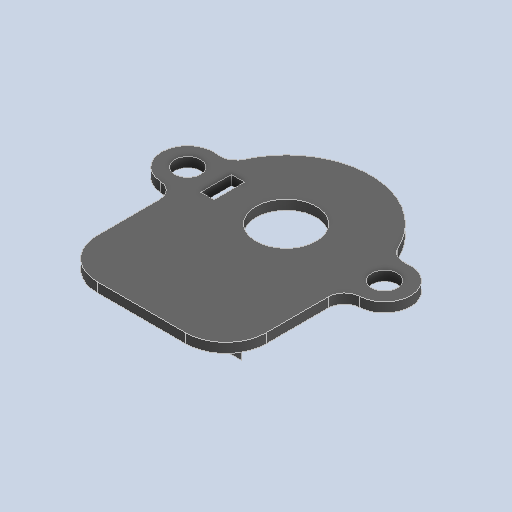
# Autodesk Inventor part: volume_case_upper
Saved by Autodesk Inventor 2026.1 (Build 301233020, 233B)
## iProperties
Created: 2026-02-01
Part Number: volume_case_upper
Material: 一般
Document SubType Name: Modeling
Designer: hibik
Density: 1 g/cm^3
Appearance: 既定
Author: hibik
Autodesk Inventor part; units mm, degrees
ref_plane "YZ Plane" through (0, 0, 0) normal (1, 0, 0) x (0, 1, 0)
ref_plane "XZ Plane" through (0, 0, 0) normal (0, 1, 0) x (-1, 0, 0)
ref_plane "XY Plane" through (0, 0, 0) normal (0, 0, 1) x (1, 0, 0)
sketch "スケッチ1" plane through (0, 0, 0) normal (0, 1, 0) x (-1, 0, 0)
  circle A0 centre (0, 0) radius 10.5
  dimension "d0" = 21
  constraints: 1 centre point, 1 coincident
  measures "d0" diameter of A0
extrude "押し出し1" add sketch "スケッチ1" along normal blind 1.2
sketch "スケッチ2" plane through (0, 1.2, 0) normal (0, 1, 0) x (1, 0, 0)
  circle A0 centre (-12.25, 0) radius 1.3 construction
  circle A1 centre (12.25, 0) radius 1.3 construction
  line L0 (15.3423, -1) -> (20.8147, -1) projected
  arc A2 (12.1791, -16.9092) -> (20.8147, -1) centre (0, 0) ccw projected
  line L1 (12.1791, -16.9092) -> (10.5, -14.0307) projected
  line L2 (10.5, -14.0307) -> (10.5, -5.244) projected
  arc A3 (12.4048, -3.2463) -> (10.5, -5.244) centre (12.5, -5.244) ccw projected
  arc A4 (12.4048, -3.2463) -> (15.3423, -1) centre (12.25, 0) ccw projected
  line L3 (9, 0) -> (9, -16.5) projected
  line L4 (-2.5, -16.5) -> (-9, -16.5) projected
  line L5 (-9, -16.5) -> (-9, 0) projected
  arc A5 (9, 0) -> (-9, 0) centre (0, 0) ccw projected
  arc A6 (15.3423, 1) -> (11.7099, 3.2048) centre (12.25, 0) ccw projected
  arc A7 (9.5571, 4.3487) -> (11.7099, 3.2048) centre (11.3776, 5.177) ccw projected
  arc A8 (9.5571, 4.3487) -> (9.333, 4.811) centre (0, 0) ccw projected
  line L6 (9.333, 4.811) -> (18.2916, 9.9833) projected
  arc A9 (20.8147, 1) -> (18.2916, 9.9833) centre (0, 0) ccw projected
  line L7 (20.8147, 1) -> (15.3423, 1) projected
  line L8 (-10.5, -5.244) -> (-10.5, -14.0307) projected
  line L9 (-12.1791, -16.9092) -> (-10.5, -14.0307) projected
  arc A10 (-20.8147, -1) -> (-12.1791, -16.9092) centre (0, 0) ccw projected
  line L10 (-15.3423, -1) -> (-20.8147, -1) projected
  arc A11 (-15.3423, -1) -> (-12.4048, -3.2463) centre (-12.25, 0) ccw projected
  arc A12 (-10.5, -5.244) -> (-12.4048, -3.2463) centre (-12.5, -5.244) ccw projected
  arc A13 (-11.7099, 3.2048) -> (-15.3423, 1) centre (-12.25, 0) ccw projected
  line L11 (-20.8147, 1) -> (-15.3423, 1) projected
  arc A14 (-18.2916, 9.9833) -> (-20.8147, 1) centre (0, 0) ccw projected
  line L12 (-9.333, 4.811) -> (-18.2916, 9.9833) projected
  arc A15 (-9.333, 4.811) -> (-9.5571, 4.3487) centre (0, 0) ccw projected
  arc A16 (-11.7099, 3.2048) -> (-9.5571, 4.3487) centre (-11.3776, 5.177) ccw projected
  line L13 (-8.1846, -18) -> (-2.5, -18) projected
  line L14 (8.1846, -18) -> (8.724, -18.9246) projected
  arc A17 (-8.724, -18.9246) -> (-2.5, -20.6882) centre (0, 0) ccw projected
  line L15 (-8.1846, -18) -> (-8.724, -18.9246) projected
  line L16 (-17.7916, 10.8493) -> (-8.833, 5.6771) projected
  arc A18 (-10.8493, 17.7916) -> (-17.7916, 10.8493) centre (0, 0) ccw projected
  line L17 (-5.6771, 8.833) -> (-10.8493, 17.7916) projected
  arc A19 (-5.6771, 8.833) -> (-8.833, 5.6771) centre (0, 0) ccw projected
  arc A20 (8.833, 5.6771) -> (5.6771, 8.833) centre (0, 0) ccw projected
  line L18 (5.6771, 8.833) -> (10.8493, 17.7916) projected
  arc A21 (17.7916, 10.8493) -> (10.8493, 17.7916) centre (0, 0) ccw projected
  line L19 (17.7916, 10.8493) -> (8.833, 5.6771) projected
  arc A22 (9.9833, 18.2916) -> (1, 20.8147) centre (0, 0) ccw projected
  line L20 (9.9833, 18.2916) -> (4.811, 9.333) projected
  arc A23 (4.811, 9.333) -> (1, 10.4523) centre (0, 0) ccw projected
  line L21 (1, 10.4523) -> (1, 20.8147) projected
  line L22 (-9.9833, 18.2916) -> (-4.811, 9.333) projected
  arc A24 (-1, 20.8147) -> (-9.9833, 18.2916) centre (0, 0) ccw projected
  line L23 (-1, 10.4523) -> (-1, 20.8147) projected
  arc A25 (-1, 10.4523) -> (-4.811, 9.333) centre (0, 0) ccw projected
  circle A26 centre (-12.25, 0) radius 3.25
  circle A27 centre (12.25, 0) radius 3.25
  line L24 (-10.5, -18) -> (10.5, -18)
  line L25 (10.5, -18) -> (10.5, -5.244)
  line L26 (10.5, -5.244) -> (-10.5, -5.244)
  line L27 (-10.5, -5.244) -> (-10.5, -18)
  circle A28 centre (-12.25, 0) radius 1.6
  circle A29 centre (12.25, 0) radius 1.6
  circle A30 centre (0, 0) radius 10.5
  arc A31 (2.5, -22.8637) -> (-2.5, -22.8637) centre (0, 0) ccw projected
  line L28 (-2.5, -22.8637) -> (-2.5, -20.6882) projected
  line L29 (-2.5, -18) -> (-2.5, -16.5) projected
  line L30 (9, -16.5) -> (2.5, -16.5) projected
  line L31 (2.5, -16.5) -> (2.5, -18) projected
  line L32 (2.5, -18) -> (8.1846, -18) projected
  arc A32 (2.5, -20.6882) -> (8.724, -18.9246) centre (0, 0) ccw projected
  line L33 (2.5, -20.6882) -> (2.5, -22.8637) projected
  point P0 (-10.4871, -0.5207)
  point P1 (-10.4871, 0.5207)
  point P2 (-9.5571, 4.3487)
  point P3 (-15.3423, -1)
  point P4 (15.3423, 1)
  point P5 (9.5571, 4.3487)
  point P6 (10.4871, 0.5207)
  point P7 (10.4871, -0.5207)
  point P8 (-11.7099, 3.2048)
  point P9 (-10.5, -5.244)
  point P10 (9.333, 4.811)
  point P11 (12.4048, -3.2463)
  point P12 (10.1939, 2.5169)
  point P13 (10.1939, -2.5169)
  point P14 (-10.1939, -2.5169)
  point P15 (-12.4048, -3.2463)
  point P16 (-10.1939, 2.5169)
  point P17 (-12.4048, -3.2463)
  point P18 (15.3423, 1)
  dimension "d3" = 3.2
  dimension "d4" = 3.2
  constraints: 8 end point, 5 coincident, 2 centre point, 2 parallel, 2 point on line, 1 horizontal, 1 perpendicular, 9 other
  measures "d3" diameter of A28
  measures "d4" diameter of A29
extrude "押し出し3" add sketch "スケッチ2" against normal up to surface (1.2 mm away) contours A4 A27 A30 A6 | A3 L26 A30 A27 | L2 L25 L24 L31 L30 L3 A30 L26 | A27 A30 A7 | L3 L30 L31 L24 L29 L4 L5 A30 | A26 A30 | L5 L4 L29 L13 L24 L27 L8 L26 A30 | A30 A26 A11 A13 | A26 A16 A30 | A30 L26 A12 A26
sketch "スケッチ3" plane through (0, 1.2, 0) normal (0, 1, 0) x (1, 0, 0)
  line L0 (-7.3, -1.4) -> (-7.3, 1.4) projected
  line L1 (-7.3, 1.4) -> (-8.5, 1.4) projected
  line L2 (-8.5, 1.4) -> (-8.5, -1.4) projected
  line L3 (-8.5, -1.4) -> (-7.3, -1.4) projected
  line L4 (-7.0857, -1.9) -> (-8.7143, -1.9)
  line L5 (-8.7143, -1.9) -> (-8.7143, 1.9)
  line L6 (-8.7143, 1.9) -> (-7.0857, 1.9)
  line L7 (-7.0857, 1.9) -> (-7.0857, -1.9)
  line L8 (-7.0857, -1.9) -> (-8.7143, 1.9) construction
  line L9 (-8.7143, -1.9) -> (-7.0857, 1.9) construction
  circle A0 centre (0, 0) radius 3.75
  point P0 (-7.9, 0)
  dimension "d9" = 0.5
  dimension "d10" = 7.5
  constraints: 12 end point, 4 point on line, 2 midpoint, 2 parallel, 1 centre point, 1 coincident, 1 horizontal, 1 perpendicular
  measures "d9" distance between parallel lines of L6 L1
  measures "d10" diameter of A0
extrude "押し出し4" cut sketch "スケッチ3" against normal through all contours L3 L2 L1 L0 | L4 L5 L6 L7 | A0
sketch "スケッチ4" plane through (0, 0, 0) normal (0, -1, 0) x (1, 0, 0)
  line L0 (-9, 16.5) -> (9, 16.5) projected
  line L1 (9, 16.5) -> (9, 10.5) projected
  line L2 (-9, 10.5) -> (-9, 16.5) projected
  line L3 (8.8, 16.3) -> (-8.8, 16.3)
  line L4 (-8.8, 16.3) -> (-8.8, 14.3)
  line L5 (-8.8, 14.3) -> (8.8, 14.3)
  line L6 (8.8, 14.3) -> (8.8, 16.3)
  point P0 (0, 0)
  point P1 (0, 14.3)
  dimension "d13" = 0.2
  dimension "d14" = 0.2
  dimension "d15" = 2
  constraints: 8 end point, 2 parallel, 1 horizontal, 1 midpoint, 1 perpendicular, 1 vertical alignment
  measures "d13" distance between parallel lines of L0 L3
  measures "d14" distance between parallel lines of L1 L6
  measures "d15" distance of L5.end L3.start
extrude "押し出し5" add sketch "スケッチ4" along normal blind 2
fillet "フィレット1" radius 5 2 edges at (10.5, 0.6, 18) (-10.5, 0.6, 18)
chamfer "面取り1" distance 2 angle 45 1 edges at (0, -2, 16.3)
